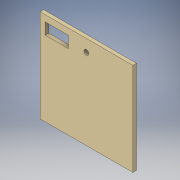
# Autodesk Inventor part: nEW bASE
Saved by Autodesk Inventor 2016 (Build 200138000, 138)
## iProperties
Created: 2017-09-12
Part Number: nEW bASE
Material: Generic
Document SubType Name: Modeling
Designer: student
Density: 1 g/cm^3
Appearance: Default
Author: student
Autodesk Inventor part; units mm, degrees
ref_plane "YZ Plane" through (0, 0, 0) normal (1, 0, 0) x (0, 1, 0)
ref_plane "XZ Plane" through (0, 0, 0) normal (0, 1, 0) x (-1, 0, 0)
ref_plane "XY Plane" through (0, 0, 0) normal (0, 0, 1) x (1, 0, 0)
sketch "Sketch1" plane through (0, 0, 0) normal (0, 0, 1) x (1, 0, 0)
  line L0 (0, 0) -> (-99.06, 0)
  line L1 (-99.06, 0) -> (-99.06, 99.06)
  line L2 (-99.06, 99.06) -> (0, 99.06)
  line L3 (0, 99.06) -> (0, 0)
  circle A0 centre (-49.53, 86.3053) radius 2.54
  line L4 (-93.595, 80.1839) -> (-68.5299, 80.1839)
  line L5 (-68.5299, 80.1839) -> (-68.5299, 92.4267)
  line L6 (-68.5299, 92.4267) -> (-93.595, 92.4267)
  line L7 (-93.595, 92.4267) -> (-93.595, 80.1839)
  dimension "d0" = 99.06
  dimension "d1" = 99.06
  dimension "d2" = 5.08
  constraints: 16 end point, 4 parallel, 2 horizontal, 2 perpendicular, 1 centre point
  measures "d0" distance of L1.end L2.end
  measures "d1" distance of L0.end L1.end
  measures "d2" diameter of A0
extrude "Extrusion1" add sketch "Sketch1" along normal blind 3.81
sketch "Sketch2" plane through (0, 0, 0) normal (0, 0, -1) x (-1, 0, 0)
  line L0 (0, 0) -> (99.06, 0) projected
  line L1 (99.06, 0) -> (99.06, 99.06) projected
  line L2 (50.116, 20.3481) -> (61.165, 20.3481)
  line L3 (61.165, 20.3481) -> (61.165, 42.3191)
  line L4 (61.165, 42.3191) -> (50.116, 42.3191)
  line L5 (50.116, 42.3191) -> (50.116, 20.3481)
  line L6 (48.9458, 20.3469) -> (37.8968, 20.3469)
  line L7 (37.8968, 20.3469) -> (37.8968, 42.3179)
  line L8 (37.8968, 42.3179) -> (48.9458, 42.3179)
  line L9 (48.9458, 42.3179) -> (48.9458, 20.3469)
  dimension "d5" = 11.049
  dimension "d6" = 21.971
  dimension "d8" = 11.049
  dimension "d9" = 21.971
  constraints: 16 end point, 4 parallel, 2 horizontal, 2 perpendicular
  measures "d5" distance of L4.end L3.end
  measures "d6" distance of L3.end L2.end
  measures "d8" distance of L7.end L8.end
  measures "d9" distance of L6.end L7.end
extrude "Extrusion2" add sketch "Sketch2" along normal blind 3.81
body "Solid1"
